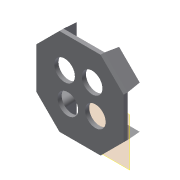
# Autodesk Inventor part: 30_Baseplate_Connector_Clamp
Saved by Autodesk Inventor 2019 (Build 230136000, 136)
## iProperties
Created: 2020-01-13
Part Number: 30_Baseplate_Connector_Clamp
Material: Generic
Document SubType Name: Modeling
Designer: diederichbenedict
Density: 1 g/cm^3
Appearance: Default
Author: diederichbenedict
Autodesk Inventor part; units mm, degrees
ref_plane "YZ Plane" through (0, 0, 0) normal (1, 0, 0) x (0, 1, 0)
ref_plane "XZ Plane" through (0, 0, 0) normal (0, 1, 0) x (-1, 0, 0)
ref_plane "XY Plane" through (0, 0, 0) normal (0, 0, 1) x (1, 0, 0)
ref_plane "Work Plane1" through (50, -100, 0) normal (0, 0, 1) x (1, 0, 0)
sketch "Sketch1" plane through (50, -100, 0) normal (0, 0, 1) x (1, 0, 0)
  line L0 (-9.1, 25) -> (-9.1, 17.5) construction
  line L1 (-9.1, 25) -> (-25, 25) construction
  line L2 (-25, 25) -> (-25, 9.1) construction
  line L3 (-17.5, 9.1) -> (-25, 9.1) construction
  line L4 (-17.5, 9.1) -> (-17.5, 15.5) construction
  arc A0 (-15.5, 17.5) -> (-17.5, 15.5) centre (-15.5, 15.5) ccw construction
  line L5 (-15.5, 17.5) -> (-9.1, 17.5) construction
  circle A1 centre (-20, 20) radius 2.2989 construction
  line L6 (-40.9, 17.5) -> (-40.9, 25)
  line L7 (-40.9, 17.5) -> (-34.5, 17.5) construction
  arc A2 (-32.5, 15.5) -> (-34.5, 17.5) centre (-34.5, 15.5) ccw construction
  line L8 (-32.5, 15.5) -> (-32.5, 9.1) construction
  line L9 (-25, 9.1) -> (-32.5, 9.1)
  line L10 (-25, 9.1) -> (-25, 25) construction
  line L11 (-25, 25) -> (-40.9, 25) construction
  circle A3 centre (-30, 20) radius 2.2989 construction
  line L12 (-40.9, 25) -> (-40.9, 32.5) construction
  line L13 (-40.9, 25) -> (-25, 25)
  line L14 (-25, 25) -> (-25, 40.9) construction
  line L15 (-32.5, 40.9) -> (-25, 40.9) construction
  line L16 (-32.5, 40.9) -> (-32.5, 34.5) construction
  arc A4 (-34.5, 32.5) -> (-32.5, 34.5) centre (-34.5, 34.5) ccw construction
  line L17 (-34.5, 32.5) -> (-40.9, 32.5) construction
  circle A5 centre (-30, 30) radius 2.2989 construction
  circle A6 centre (-20, 30) radius 2.2989 construction
  line L18 (-25, 40.9) -> (-17.5, 40.9) construction
  line L19 (-25, 40.9) -> (-25, 25) construction
  line L20 (-25, 25) -> (-9.1, 25) construction
  line L21 (-9.1, 32.5) -> (-9.1, 25) construction
  line L22 (-9.1, 32.5) -> (-15.5, 32.5) construction
  arc A7 (-17.5, 34.5) -> (-15.5, 32.5) centre (-15.5, 34.5) ccw construction
  line L23 (-17.5, 34.5) -> (-17.5, 40.9) construction
  line L24 (-25, 9.1) -> (-32.5, 9.1)
  line L25 (-40.9, 17.5) -> (-32.5, 9.1)
  line L26 (-40.9, 17.5) -> (-40.9, 25)
  line L27 (-25, 25) -> (-40.9, 25)
  line L28 (-25, 9.1) -> (-25, 25)
  arc A8 (-32.5755, 19.3934) -> (-26.2755, 19.3934) centre (-29.4255, 19.3934) ccw projected
  circle A9 centre (-29.4255, 19.3934) radius 3.75
  line L29 (-40.9, 17.5) -> (-40.9, 25) projected
  line L30 (-25, 9.1) -> (-32.5, 9.1) projected
  line L31 (-40.9, 25) -> (-25, 25) projected
  point P0 (-50, 100)
  dimension "d0" = 7.5
  constraints: 16 end point, 3 collinear, 1 centre point, 1 coincident
  measures "d0" diameter of A9
extrude "Extrusion1" add sketch "Sketch1" along normal blind 1.5
sketch "Sketch2" plane through (50, -100, 0) normal (0, 0, -1) x (-1, 0, 0)
  circle A0 centre (29.4255, 19.3934) radius 3.75 projected
  line L0 (25, 25) -> (40.9, 25) projected
  line L1 (25, 9.1) -> (25, 25) projected
  line L2 (32.5, 9.1) -> (25, 9.1) projected
  line L3 (40.9, 17.5) -> (32.5, 9.1) projected
  line L4 (40.9, 25) -> (40.9, 17.5) projected
  line L5 (32.5, -15.5) -> (32.5, 15.5) projected
  arc A1 (34.5, 17.5) -> (32.5, 15.5) centre (34.5, 15.5) ccw projected
  line L6 (34.5, 17.5) -> (65.5, 17.5) projected
  line L7 (65.4275, 17.6356) -> (34.5, 17.6356)
  arc A2 (34.5, 17.6356) -> (32.3644, 15.5) centre (34.5, 15.5) ccw
  line L8 (32.3644, 15.5) -> (32.3644, -15.5)
  line L9 (40.9, 17.5) -> (32.5, 9.1) projected
  point P0 (50, 100)
  point P1 (41.0356, 17.6356)
  point P2 (32.3644, 8.9644)
  constraints: 4 end point, 4 point on line, 2 point on circle, 1 centre point, 2 other
extrude "Extrusion2" add sketch "Sketch2" along normal blind 5 draft -3 contours L3 L5 A1 L6
pattern_circular "Circular Pattern1" count 4 over 360 about axis through (25, -75, 0) along (0, 0, 1) of "Extrusion1", "Extrusion2"
body "Solid1"
